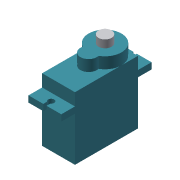
# Autodesk Inventor part: Mikroservo
Saved by Autodesk Inventor 2015 (Build 190159000, 159)
## iProperties
Created: 2015-02-07
Part Number: Mikroservo
Material: ABS-Kunststoff
Document SubType Name: Modeling
Designer: Luki
Density: 1.06 g/cm^3
Appearance: Kadettenblau
Author: Luki
Autodesk Inventor part; units mm, degrees
ref_plane "YZ Plane" through (0, 0, 0) normal (1, 0, 0) x (0, 1, 0)
ref_plane "XZ Plane" through (0, 0, 0) normal (0, 1, 0) x (-1, 0, 0)
ref_plane "XY Plane" through (0, 0, 0) normal (0, 0, 1) x (1, 0, 0)
sketch "Skizze1" plane through (0, 0, 0) normal (0, 0, 1) x (1, 0, 0)
  line L0 (0, 16.1) -> (0, -16.1) projected
  line L1 (-8.4, 0) -> (8.4, 0) projected
  line L2 (-6, -11.5) -> (6, -11.5)
  line L3 (6, -11.5) -> (6, 11.5)
  line L4 (6, 11.5) -> (-6, 11.5)
  line L5 (-6, 11.5) -> (-6, -11.5)
  line L6 (-6, -11.5) -> (6, 11.5) construction
  line L7 (6, -11.5) -> (-6, 11.5) construction
  point P0 (0, 0)
  dimension "d0" = 12
  dimension "d1" = 23
  constraints: 12 end point, 2 midpoint, 2 parallel, 1 horizontal, 1 perpendicular
  measures "d0" distance between parallel lines of L5 L3
  measures "d1" distance between parallel lines of L4 L2
extrude "Extrusion1" add sketch "Skizze1" along normal blind 16.2
sketch "Skizze2" plane through (0, 0, 16.2) normal (0, 0, 1) x (1, 0, 0)
  line L0 (-6, -11.5) -> (-6, 11.5) projected
  line L1 (-6, 11.5) -> (6, 11.5) projected
  line L2 (6, 11.5) -> (6, -11.5) projected
  line L3 (6, -11.5) -> (-6, -11.5) projected
  line L4 (6, 11.5) -> (-6, 11.5)
  line L5 (-6, 11.5) -> (-6, 16.5)
  line L6 (-6, 16.5) -> (6, 16.5)
  line L7 (6, 16.5) -> (6, 11.5)
  line L8 (-6, -11.5) -> (6, -11.5)
  line L9 (6, -11.5) -> (6, -16.5)
  line L10 (6, -16.5) -> (-6, -16.5)
  line L11 (-6, -16.5) -> (-6, -11.5)
  line L12 (-6, 11.5) -> (-6, -11.5) projected
  point P0 (0, 0)
  dimension "d4" = 5
  dimension "d5" = 5
  constraints: 16 end point, 4 parallel, 2 horizontal, 2 perpendicular, 2 point on line
  measures "d4" distance between parallel lines of L3 L10
  measures "d5" distance between parallel lines of L1 L6
extrude "Extrusion2" add sketch "Skizze2" along normal blind 2.3
sketch "Skizze3" plane through (0, 0, 18.5) normal (0, 0, 1) x (1, 0, 0)
  line L0 (6, -16.5) -> (-6, -16.5) projected
  line L1 (-6, -16.5) -> (-6, 16.5) projected
  line L2 (-6, 16.5) -> (6, 16.5) projected
  line L3 (6, 16.5) -> (6, -16.5) projected
  line L4 (-6, -11.5) -> (6, -11.5)
  line L5 (6, -11.5) -> (6, 11.5)
  line L6 (6, 11.5) -> (-6, 11.5)
  line L7 (-6, 11.5) -> (-6, -11.5)
  line L8 (-6, -11.5) -> (6, 11.5) construction
  line L9 (6, -11.5) -> (-6, 11.5) construction
  point P0 (0, 0)
  dimension "d8" = 11.5
  constraints: 12 end point, 2 midpoint, 2 parallel, 1 horizontal, 1 perpendicular, 1 point on line
  measures "d8" distance from line of L6 point (0, 0)
extrude "Extrusion3" add sketch "Skizze3" along normal blind 4.5 contours L4 L1 L6 L3
sketch "Skizze4" plane through (0, 0, 23) normal (0, 0, 1) x (1, 0, 0)
  line L0 (-6, 11.5) -> (6, 11.5) projected
  line L1 (6, 11.5) -> (6, -11.5) projected
  line L2 (6, -11.5) -> (-6, -11.5) projected
  line L3 (-6, -11.5) -> (-6, 11.5) projected
  line L4 (6, 16.5) -> (-6, 16.5) projected
  line L5 (-6, 16.5) -> (-6, 11.5) projected
  line L6 (6, 11.5) -> (6, 16.5) projected
  line L7 (6, -16.5) -> (6, -11.5) projected
  line L8 (-6, -16.5) -> (6, -16.5) projected
  line L9 (-6, -11.5) -> (-6, -16.5) projected
  line L10 (-8.4, 0) -> (8.4, 0) projected
  line L11 (0, 23.1) -> (0, -23.1) projected
  circle A0 centre (0, 5.5) radius 6
  circle A1 centre (0, -0.5) radius 3
  point P0 (0, 0)
  dimension "d11" = 11
  dimension "d12" = 12
  dimension "d13" = 17
  dimension "d14" = 6
  constraints: 2 centre point, 2 point on line
  measures "d11" distance from line of L4 A0.centre
  measures "d12" diameter of A0
  measures "d13" distance from line of L4 A1.centre
  measures "d14" diameter of A1
extrude "Extrusion4" add sketch "Skizze4" along normal blind 4.1 contours A0 A1 L11 | L11 A1 A0 | A1 A0 L10 L11 | L11 L10 A0 A1 | A0 L10 A1 | L11 A0 L10 | L10 A0 L11 | A1 L10 A0 | L10 A0 L11 A1 | L10 A1 L11 A0
sketch "Skizze5" plane through (0, 0, 27.1) normal (0, 0, 1) x (1, 0, 0)
  arc A0 (2.9047, 0.25) -> (-2.9047, 0.25) centre (0, 5.5) ccw projected
  arc A1 (-2.9047, 0.25) -> (2.9047, 0.25) centre (0, -0.5) ccw projected
  circle A2 centre (0, 5.5) radius 2.4
  point P0 (0, 0)
  dimension "d17" = 4.8
  constraints: 1 centre point, 1 coincident
  measures "d17" diameter of A2
extrude "Extrusion5" add sketch "Skizze5" along normal blind 2.8 contours A2
sketch "Skizze6" plane through (0, 0, 18.5) normal (0, 0, 1) x (1, 0, 0)
  line L0 (6, -16.5) -> (-6, -16.5) projected
  line L1 (-6, -16.5) -> (-6, -11.5) projected
  line L2 (6, -11.5) -> (-6, -11.5) projected
  line L3 (6, 11.5) -> (6, -11.5) projected
  line L4 (-6, 11.5) -> (6, 11.5) projected
  line L5 (-6, 11.5) -> (-6, 16.5) projected
  line L6 (-6, 16.5) -> (6, 16.5) projected
  line L7 (6, 16.5) -> (6, 11.5) projected
  line L8 (6, -11.5) -> (6, -16.5) projected
  line L9 (-6, -11.5) -> (-6, 11.5) projected
  line L10 (0, 23.1) -> (0, -23.1) projected
  circle A0 centre (0, 14.2) radius 1.1
  line L11 (6, 16.5) -> (-6, 16.5) projected
  line L12 (0.6, 14.1) -> (-0.6, 14.1)
  line L13 (-0.6, 14.1) -> (-0.6, 16.5)
  line L14 (-0.6, 16.5) -> (0.6, 16.5)
  line L15 (0.6, 16.5) -> (0.6, 14.1)
  line L16 (0.6, 14.1) -> (-0.6, 16.5) construction
  line L17 (-0.6, 14.1) -> (0.6, 16.5) construction
  point P0 (0, 0)
  point P1 (0, 15.3)
  dimension "d21" = 2.2
  dimension "d20" = 2.3
  dimension "d22" = 1.2
  constraints: 12 end point, 3 point on line, 2 midpoint, 2 parallel, 1 horizontal, 1 perpendicular, 1 vertical alignment, 2 other
  measures "d20" distance from line of L6 point (0, 14.2)
  measures "d22" distance between parallel lines of L15 L13
extrude "Extrusion6" cut sketch "Skizze6" against normal blind 2.8 contours A0 L13 L12 L10 | L10 L12 L15 A0 | L15 A0 L10 L6 | L12 L13 A0 L10 | L10 A0 L15 L12 | L13 L6 L10 A0
mirror "Spiegeln1" about plane through (0, 0, 0) normal (0, 1, 0) of "Extrusion6"
